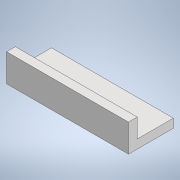
# Autodesk Inventor part: Part17
Saved by Autodesk Inventor 2022 (Build 260153000, 153)
## iProperties
Created: 2022-06-07
Part Number: Part17
Material: Generic
Document SubType Name: Modeling
Designer: tecware
Density: 1 g/cm^3
Appearance: Default
Author: tecware
Autodesk Inventor part; units mm, degrees
ref_plane "YZ Plane" through (0, 0, 0) normal (1, 0, 0) x (0, 1, 0)
ref_plane "XZ Plane" through (0, 0, 0) normal (0, 1, 0) x (-1, 0, 0)
ref_plane "XY Plane" through (0, 0, 0) normal (0, 0, 1) x (1, 0, 0)
sketch "Sketch1" plane through (0, 0, 0) normal (0, 0, 1) x (1, 0, 0)
  line L0 (2.2815, -0.606) -> (30.1037, -0.606)
  line L1 (30.1037, -0.606) -> (30.1037, -4.956)
  line L2 (30.1037, -4.956) -> (2.2815, -4.956)
  line L3 (2.2815, -4.956) -> (2.2815, -0.606)
  point P0 (0, 0)
  dimension "d1" = 4.35
  dimension "d2" = 27.8222
  constraints: 8 end point, 4 parallel, 1 perpendicular
  measures "d1" distance of L2.end L0.start
  measures "d2" distance of L0.start L0.end
extrude "Extrusion1" add sketch "Sketch1" along normal blind 2
sketch "Sketch2" plane through (0, 0, 0) normal (0, 0, -1) x (-1, 0, 0)
  line L0 (-2.2815, -4.956) -> (-30.1037, -4.956) projected
  line L1 (-30.1037, -4.956) -> (-30.1037, -0.606) projected
  line L2 (-2.2815, -4.956) -> (-30.1037, -4.956)
  line L3 (-30.1037, -4.956) -> (-30.1037, -2.956)
  line L4 (-30.1037, -2.956) -> (-2.2815, -2.956)
  line L5 (-2.2815, -2.956) -> (-2.2815, -4.956)
  point P0 (0, 0)
  dimension "d5" = 2
  constraints: 8 end point, 1 point on line
  measures "d5" distance of L2.end L3.end
extrude "Extrusion2" add sketch "Sketch2" along normal blind 17.6
chamfer "Chamfer1" distance 1 angle 45 1 edges at (16.1926, -2.956, -17.6)
body "Solid1"
